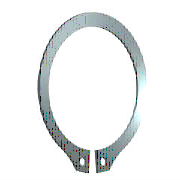
# Autodesk Inventor part: DIN 471 - 10x1
Saved by Autodesk Inventor 2022 (Build 260153000, 153)
## iProperties
Created: 2017-02-09
Part Number: DIN 471 - 10x1
Material: Acero, suave
Description: Anillas de retención para el eje
Document SubType Name: Modeling
Standard: DIN 471
Designer: Cristiano
Standard Revision: 2011-04
Standards Organization: DIN
Language: es-ES
Size Designation: 10x1
Categories: <MemberInstance><Categories><Category DisplayName="Piezas del eje" InternalName="7f7aeb1f-a693-4053-b835-cee3144e0d98" Mnemonic="SHFT"><Category DisplayName="Arandelas elásticas de retención" InternalName="413b042a-1f46-4051-a560-0e0e417af91f" Mnemonic="CLIP"><CategoryParameter DisplayName="Grosor" InternalName="230c7f7c-2544-4c6d-b8d5-773e831b23fa" Mnemonic="thick"/><CategoryParameter DisplayName="Diámetro del acanalado" InternalName="4054b45c-161d-4ad6-befb-f30b3855ce84" Mnemonic="grvdia"/><CategoryParameter DisplayName="Anchura del acanalado" InternalName="4dde6996-4bf1-443b-8317-d4f4fc6b9be0" Mnemonic="NB"/><CategoryParameter DisplayName="Diámetro de eje" InternalName="a433c9ab-b9eb-4798-a453-f2210a67728e" Mnemonic="shaftdia"/><Category DisplayName="Externo/a" InternalName="a9a2b132-a8be-48ab-9c3d-0c324a909558" Mnemonic="OUCLIP"><CategoryParameter DisplayName="Diámetro mín. de eje" InternalName="62b77b9b-1e86-4b9a-9911-d7c0fa48fc9a" Mnemonic="shaftdiamin"/><CategoryParameter DisplayName="Diámetro exterior" InternalName="a3599e7b-be7c-41b5-9a50-6dab253b0906" Mnemonic="outdia"/></Category></Category></Category><Category DisplayName="TipoDatos" InternalName="23b78d0f-2648-40c6-8793-ca6db495c9e8" Mnemonic="DATATYPE"><CategoryParameter DisplayName="NombreVisualización" InternalName="05415f3d-3907-474b-a020-eb9d644f4cf3" Mnemonic="DISPLAYNAME"/><CategoryParameter DisplayName="Estándar" InternalName="0c0a119c-1e12-4c84-803f-101930972f5e" Mnemonic="STANDARD"/><CategoryParameter DisplayName="Descripción" InternalName="13903e3d-64b1-4950-80da-f627842ea37f" Mnemonic="DESCRIPTION"/><CategoryParameter DisplayName="Designación" InternalName="2675968c-4ce5-49e0-a4f5-552d29089031" Mnemonic="DESIGNATION"/><CategoryParameter DisplayName="Fila por defecto" InternalName="2af9ec52-faaa-4026-b378-f9fa4afca842" Mnemonic="DEFAULTROW"/><CategoryParameter DisplayName="Nombre de carpeta" InternalName="3f06958e-8713-4116-9be7-ed6184ecc97b" Mnemonic="FOLDERNAME"/><CategoryParameter DisplayName="Guid de revisión" InternalName="45a75005-10b1-4dfc-8d6d-dfe629f0b93c" Mnemonic="REVISIONGUID"/><CategoryParameter DisplayName="NombreArchivo" InternalName="8b46a4cc-9585-4fed-90c3-899f57e09a73" Mnemonic="FILENAME"/><CategoryParameter DisplayName="OrgEstand" InternalName="8f5914e1-4693-403f-8ab5-d37768198c9d" Mnemonic="STDSORG"/><CategoryParameter DisplayName="Versión de familia" InternalName="914462f6-6e19-4b14-ba84-155b9680b1d0" Mnemonic="FAMILYREVISION"/><CategoryParameter DisplayName="Revisión de Norma" InternalName="91d5a463-65c2-4fde-b823-3b7fea5e8e17" Mnemonic="STANDARDREVISION"/><CategoryParameter DisplayName="Revisión del miembro" InternalName="a65d44b9-392f-4f4f-857b-e4b3d54996fe" Mnemonic="MEMBERREVISION"/><CategoryParameter DisplayName="FormatoDelimitación" InternalName="bc51e27b-3422-4e78-93ef-cec197ddf230" Mnemonic="CLIPFORMAT"/><CategoryParameter DisplayName="Fabricante" InternalName="cd6c7a72-a28a-4e50-99a9-2c7f4e13e5ad" Mnemonic="MANUFACTURER"/><CategoryParameter DisplayName="NombreInterno" InternalName="cf1d0246-76d9-4b4a-8305-fa0409afb5c1" Mnemonic="INTERNALNAME"/><CategoryParameter DisplayName="EsMétrico" InternalName="e2385c5b-1ea4-4823-96a8-8de651266ec3" Mnemonic="ISMETRIC"/><Category DisplayName="Pieza" InternalName="c0e0b642-3bcb-4cc8-9e80-f96d35c4afa4" Mnemonic="PART"><CategoryParameter DisplayName="Número de pieza" InternalName="016b6077-bfbe-49bd-92c9-d8d59c39c941" Mnemonic="PARTNUMBER"/><CategoryParameter DisplayName="Referencia de almacén" InternalName="4dba7c1c-e26c-444e-836c-b08b433409a8" Mnemonic="STOCKNUMBER"/><CategoryParameter DisplayName="Clave de material" InternalName="5c9a8adb-dd2b-4535-b97f-0a94a95fe41f" Mnemonic="MATERIALKEY"/><CategoryParameter DisplayName="Material" InternalName="818a152a-d3c3-49ca-80ee-df7d91421b8e" Mnemonic="MATERIAL"/></Category></Category><Category DisplayName="Asignación de elementos heredados DA" InternalName="924fff40-ddd0-4eff-ad42-30e3774ef79e" Mnemonic="LEGACYMAPDA"><CategoryParameter DisplayName="DACookie" InternalName="316934ee-8fe1-4c7a-9c36-f2d79e1add1a" Mnemonic="DACOOKIE"/></Category></Categories><FamilyTemplate Id="D471A"><FamilyTemplateParameters><FamilyTemplateParameter ObjectType="kUserParameterObject" ValueType="xs:double" Id="2" ObjectReferenceKey="Diam2"/><FamilyTemplateParameter ObjectType="kUserParameterObject" ValueType="xs:double" Id="5" ObjectReferenceKey="Diam5"/><FamilyTemplateParameter ObjectType="kUserParameterObject" ValueType="xs:double" Id="6" ObjectReferenceKey="ParA"/><FamilyTemplateParameter ObjectType="kUserParameterObject" ValueType="xs:double" Id="7" ObjectReferenceKey="b"/><FamilyTemplateParameter ObjectType="kUserParameterObject" ValueType="xs:double" Id="8" ObjectReferenceKey="ParS"/><FamilyTemplateParameter ObjectType="kUserParameterObject" ValueType="xs:string" Id="118" ObjectReferenceKey="TEMPLATE"/><FamilyTemplateParameter ObjectType="kPropertyObject" ValueType="xs:string" Id="100" ObjectReferenceKey="{32853F0F-3444-11d1-9E93-0060B03C1CA6}" SubObjectId="52"/><FamilyTemplateParameter ObjectType="kPropertyObject" ValueType="xs:string" Id="105" ObjectReferenceKey="{32853F0F-3444-11d1-9E93-0060B03C1CA6}" SubObjectId="5"/><FamilyTemplateParameter ObjectType="kPartComponentDefinitionObject" ValueType="xs:string" Id="110" SubObjectId="Material"/></FamilyTemplateParameters></FamilyTemplate><CategoryParameterMap><ParamToTemplateMap><ParamToTemplate CategoryParameter="//CategoryParameter[@InternalName='05415f3d-3907-474b-a020-eb9d644f4cf3']" ConstantValue="DIN 471"/><ParamToTemplate CategoryParameter="//CategoryParameter[@InternalName='cf1d0246-76d9-4b4a-8305-fa0409afb5c1']" ConstantValue="0A5383B2-1225-43D6-9D10-35CDC30ECC55"/><ParamToTemplate CategoryParameter="//CategoryParameter[@InternalName='3f06958e-8713-4116-9be7-ed6184ecc97b']" ConstantValue="DIN 471(1)"/><ParamToTemplate CategoryParameter="//CategoryParameter[@InternalName='914462f6-6e19-4b14-ba84-155b9680b1d0']" ConstantValue="10"/><ParamToTemplate CategoryParameter="//CategoryParameter[@InternalName='bc51e27b-3422-4e78-93ef-cec197ddf230']" ConstantValue="CF_INVENTOR.STDPARTS"/><ParamToTemplate CategoryParameter="//CategoryParameter[@InternalName='e2385c5b-1ea4-4823-96a8-8de651266ec3']" ConstantValue="true"/><ParamToTemplate CategoryParameter="//CategoryParameter[@InternalName='13903e3d-64b1-4950-80da-f627842ea37f']" ConstantValue="Retaining rings for shaft"/><ParamToTemplate CategoryParameter="//CategoryParameter[@InternalName='8f5914e1-4693-403f-8ab5-d37768198c9d']" ConstantValue="DIN"/><ParamToTemplate CategoryParameter="//CategoryParameter[@InternalName='0c0a119c-1e12-4c84-803f-101930972f5e']" ConstantValue="DIN 471"/><ParamToTemplate CategoryParameter="//CategoryParameter[@InternalName='cd6c7a72-a28a-4e50-99a9-2c7f4e13e5ad']" TemplateParameter="104"/><ParamToTemplate CategoryParameter="//CategoryParameter[@InternalName='91d5a463-65c2-4fde-b823-3b7fea5e8e17']" ConstantValue="2011-04"/><ParamToTemplate CategoryParameter="//CategoryParameter[@InternalName='45a75005-10b1-4dfc-8d6d-dfe629f0b93c']" ConstantValue="ec345a03-b14a-4139-81b0-79cb3bd95a4f"/><ParamToTemplate CategoryParameter="//CategoryParameter[@InternalName='2af9ec52-faaa-4026-b378-f9fa4afca842']" ConstantValue="10"/><ParamToTemplate CategoryParameter="//CategoryParameter[@InternalName='8b46a4cc-9585-4fed-90c3-899f57e09a73']" ConstantValue="DIN 471 - 10x1"/><ParamToTemplate CategoryParameter="//CategoryParameter[@InternalName='a65d44b9-392f-4f4f-857b-e4b3d54996fe']" ConstantValue="15972ff6-e41f-4cce-a93d-92190bb39967"/><ParamToTemplate CategoryParameter="//CategoryParameter[@InternalName='a433c9ab-b9eb-4798-a453-f2210a67728e']" ConstantValue="10"/><ParamToTemplate CategoryParameter="//CategoryParameter[@InternalName='4dde6996-4bf1-443b-8317-d4f4fc6b9be0']" ConstantValue="1,1"/><ParamToTemplate CategoryParameter="//CategoryParameter[@InternalName='316934ee-8fe1-4c7a-9c36-f2d79e1add1a']" ConstantValue="*DIN~D471~10x1*"/><ParamToTemplate CategoryParameter="//CategoryParameter[@InternalName='2675968c-4ce5-49e0-a4f5-552d29089031']" TemplateParameter="100"/><ParamToTemplate CategoryParameter="//CategoryParameter[@InternalName='4054b45c-161d-4ad6-befb-f30b3855ce84']" TemplateParameter="2"/><ParamToTemplate CategoryParameter="//CategoryParameter[@InternalName='818a152a-d3c3-49ca-80ee-df7d91421b8e']" TemplateParameter="110"/><ParamToTemplate CategoryParameter="//CategoryParameter[@InternalName='016b6077-bfbe-49bd-92c9-d8d59c39c941']" TemplateParameter="105"/><ParamToTemplate CategoryParameter="//CategoryParameter[@InternalName='230c7f7c-2544-4c6d-b8d5-773e831b23fa']" TemplateParameter="8"/></ParamToTemplateMap></CategoryParameterMap></MemberInstance>
Density: 7.85 g/cm^3
Appearance: Semipulido
IsCustomPart: 0
Author: Cristiano
Autodesk Inventor part; units mm, degrees
note: some values were not read from the file. Left out: dimensions or parameters whose unit could not be read.
ref_plane "WorkPlane1" through (0, 0, 0) normal (0, 0, 1) x (1, 0, 0)
ref_plane "Work Plane2" through (0, 0, -1) normal (0, 0, 1) x (1, 0, 0)
ref_plane "WorkPlane2" through (0, 0, 1.5) normal (0, 0, 1) x (1, 0, 0)
sketch "Boceto1" plane through (0, 0, 0) normal (0, 0, 1) x (1, 0, 0)
  point P0 (0, 0)
sketch "Boceto2" plane through (0, 0, 0) normal (0, 0, 1) x (1, 0, 0)
  line L0 (3.75, -7.5121) -> (3.75, -4.65)
  line L1 (0.75, -8.041) -> (3.75, -7.5121)
  line L2 (0.75, -4.741) -> (0.75, -8.041)
  arc A0 (0.75, -4.741) -> (-0.75, -4.741) centre (0, 0) ccw
  line L3 (-0.75, -4.741) -> (-0.75, -8.041)
  line L4 (-0.75, -8.041) -> (-3.75, -7.5121)
  line L5 (-3.75, -7.5121) -> (-3.75, -4.65)
  arc A1 (3.75, -4.65) -> (-3.75, -4.65) centre (0, 0.35) ccw
  dimension "d2" = 4.8
  dimension "d4" = 6.25
  dimension "d6" = 0
  dimension "d8" = 0.75
  dimension "d10" = 0.75
  dimension "d12" = 3.3
  dimension "d14" = 3.3
  dimension "d16" = 80
  dimension "d18" = 80
  dimension "d20" = 3
  dimension "d22" = 3
  dimension "d24" = 0.35
  dimension "d52" = 0
  dimension "d53" = 0
  constraints: 12 end point, 4 point on circle, 4 vertical, 2 centre point
  measures "d2" radius of A0
  measures "d4" radius of A1
  measures "d6" horizontal distance of A1.centre A0.centre
  measures "d8" horizontal distance of L2.start A0.centre
  measures "d10" horizontal distance of L3.start A0.centre
  measures "d12" distance of L3.start L3.end
  measures "d14" distance of L2.start L1.start
  measures "d16" angle of L1 L2
  measures "d18" angle of L3 L4
  measures "d20" horizontal distance of L3.start L5.end
  measures "d22" horizontal distance of L0.start L2.start
  measures "d24" distance of A0.centre A1.centre
  measures "d52" distance of point (0, 0) A0.centre
  measures "d53" distance of A0.centre point (0, 0)
extrude "Extrusión1" add sketch "Boceto2" along normal blind 1
sketch "Boceto3" plane through (0, 0, 1) normal (0, 0, 1) x (1, 0, 0)
  line L0 (-0.75, -4.741) -> (-0.75, -8.041) projected
  line L1 (-0.75, -8.041) -> (-3.75, -7.5121) projected
  point P0 (-1.95, -6.3215)
  dimension "d30" = 1.2
  dimension "d32" = 1.485
  measures "d30" distance from line of L0 point (-1.95, -6.322)
  measures "d32" distance from line of L1 point (-1.95, -6.322)
hole "Agujero1" at (-1.95, -6.3215, 1) direction (0, 0, -1) diameter 1.5 end through all
sketch "Boceto4" plane through (0, 0, 1) normal (0, 0, 1) x (1, 0, 0)
  line L0 (0.75, -8.041) -> (0.75, -4.741) projected
  line L1 (3.75, -7.5121) -> (0.75, -8.041) projected
  point P0 (1.95, -6.3215)
  dimension "d41" = 1.2
  dimension "d43" = 1.485
  measures "d41" distance from line of L0 point (1.95, -6.322)
  measures "d43" distance from line of L1 point (1.95, -6.322)
hole "Agujero2" at (1.95, -6.3215, 1) direction (0, 0, -1) diameter 1.5 end through all
fillet "Empalme1" radius 2.25 2 edges at (-3.75, -7.5121, 0.5) (3.75, -7.5121, 0.5)
equation "\"d2\" = 0.5 * Diam2"
equation "\"d4\" = 0.166667 * ParA + 0.5 * Diam2 + 0.5 * b"
equation "\"d8\" = 0.5 * Diam5"
equation "\"d10\" = 0.5 * Diam5"
equation "\"d12\" = ParA"
equation "\"d14\" = ParA"
equation "\"d20\" = 2 * Diam5"
equation "\"d22\" = 2 * Diam5"
equation "\"d24\" = -msp_r2 + 0.5 * Diam2 + b"
equation "\"d25\" = ParS"
equation "\"d30\" = 0.8 * Diam5"
equation "\"d32\" = 0.45 * ParA"
equation "\"d33\" = Diam5"
equation "\"d41\" = 0.8 * Diam5"
equation "\"d43\" = 0.45 * ParA"
equation "\"d44\" = Diam5"
equation "\"d51\" = 1.5 * Diam5"
equation "\"Diam5\" = 1.5"
equation "\"ParA\" = 3.3"
equation "\"ParS\" = 1"
equation "\"Diam2\" = 9.6"
equation "\"msp_r2\" = 0.166667 * ParA + 0.5 * Diam2 + 0.5 * b"
equation "\"TEMPLATE\" = 1.2345"
body "Solid1"
